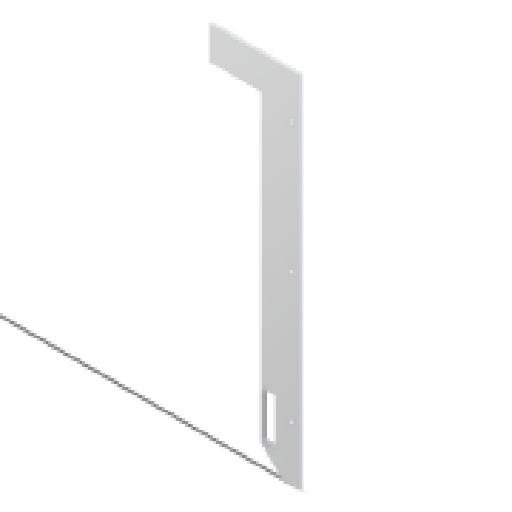
# Autodesk Inventor part: Drag Chain Cover Panel
Saved by Autodesk Inventor 2023.2 (Build 272271000, 271)
## iProperties
Created: 2023-02-24
Part Number: Drag Chain Cover Panel
Material: Aluminum 6061
Document SubType Name: Modeling
Designer: remop
Density: 2.7 g/cm^3
Appearance: Aluminum - Flat
Author: remop
Autodesk Inventor part; units mm, degrees
ref_plane "YZ Plane" through (0, 0, 0) normal (1, 0, 0) x (0, 1, 0)
ref_plane "XZ Plane" through (0, 0, 0) normal (0, 1, 0) x (-1, 0, 0)
ref_plane "XY Plane" through (0, 0, 0) normal (0, 0, 1) x (1, 0, 0)
sketch "Sketch1" plane through (0, 0, 0) normal (0, 0, 1) x (1, 0, 0)
  line L0 (-209.6812, -263.8586) -> (-209.6812, -8.8159) projected
  arc A0 (-209.6812, -8.8159) -> (-193.9694, 2.087) centre (-210.1812, 8.6769) ccw projected
  line L1 (-193.9694, 2.087) -> (-181.7072, 32.2534) projected
  arc A1 (-181.7072, 32.2534) -> (-181.1183, 35.2659) centre (-189.1183, 35.2659) ccw projected
  line L2 (-181.1183, 35.2659) -> (-181.1183, 96.1414) projected
  line L3 (-181.1183, 96.1414) -> (-26.7601, 96.1414) projected
  line L4 (-26.7601, 96.1414) -> (-26.7601, -154.4598) projected
  line L5 (-26.7601, -154.4598) -> (-51.6589, -154.4598) projected
  arc A2 (-51.6589, -154.4598) -> (-66.1514, -181.7688) centre (-51.6589, -171.9598) ccw projected
  line L6 (-66.1514, -181.7688) -> (-37.4983, -224.1032) projected
  line L7 (-37.4983, -224.1032) -> (-37.4983, -263.8586) projected
  line L8 (-37.4983, -263.8586) -> (-209.6812, -263.8586) projected
  circle A3 centre (-14.2602, -188.2205) radius 1.4 projected
  circle A4 centre (7.7398, -188.2205) radius 1.4 projected
  circle A5 centre (-3.2602, -180.2205) radius 1.4 projected
  line L9 (38.5068, -227.443) -> (38.5068, -237.331) projected
  line L10 (38.5068, -237.331) -> (14.3647, -261.4731) projected
  line L11 (14.3647, -261.4731) -> (4.4767, -261.4731) projected
  line L12 (4.4767, -261.4731) -> (-26.5537, -230.4427) projected
  arc A6 (-26.9169, -230.0029) -> (-26.5537, -230.4427) centre (-24.4324, -228.3213) ccw projected
  line L13 (-26.9169, -230.0029) -> (-61.6727, -178.6518) projected
  arc A7 (-44.3145, -161.2936) -> (-61.6727, -178.6518) centre (-51.3209, -171.6454) ccw projected
  line L14 (-44.3145, -161.2936) -> (-22.2602, -176.2205) projected
  line L15 (-22.2602, -176.2205) -> (15.7398, -176.2205) projected
  line L16 (15.7398, -176.2205) -> (15.7398, -204.6759) projected
  line L17 (15.7398, -204.6759) -> (38.5068, -227.443) projected
  circle A8 centre (21.8647, -223.6177) radius 4 projected
  circle A9 centre (0.6515, -202.4045) radius 4 projected
  circle A10 centre (-20.5617, -223.6177) radius 4 projected
  circle A11 centre (0.6515, -244.831) radius 4 projected
  circle A12 centre (0.6515, -223.6177) radius 13 projected
  line L18 (55.2634, 96.1414) -> (55.2634, -263.8586) projected
  line L19 (40.2634, 96.1414) -> (-459.7366, 96.1414) projected
  line L20 (40.2634, 96.1414) -> (55.2634, 96.1414)
  line L21 (20.2634, 66.0678) -> (-26.7366, 66.0678) projected
  line L22 (20.2634, -173.9322) -> (20.2634, 66.0678) projected
  line L23 (20.2634, -173.9322) -> (20.2634, -206.3712)
  line L24 (20.2634, -206.3712) -> (40.2634, -226.3712)
  line L25 (40.2634, -226.3712) -> (55.2634, -226.3712)
  line L26 (-25.7601, 66.0678) -> (-25.7601, 96.1414)
  circle A13 centre (-71.7601, 91.1414) radius 1.45 projected
  circle A14 centre (-41.7601, 91.1414) radius 1.45 projected
  circle A15 centre (-66.4329, -190.3739) radius 1.45 projected
  circle A16 centre (-46.6589, -149.4598) radius 1.45 projected
  circle A17 centre (-195.1812, -258.8586) radius 1.45 projected
  circle A18 centre (-174.1183, 35.2659) radius 1.45 projected
  line L27 (-48.8209, -179.8954) -> (-45.8209, -179.8954) projected
  line L28 (-45.8209, -179.8954) -> (-45.8209, -163.3954) projected
  line L29 (-45.8209, -163.3954) -> (-48.8209, -163.3954) projected
  line L30 (-48.8209, -163.3954) -> (-48.8209, -179.8954) projected
  line L31 (-56.8209, -179.8954) -> (-53.8209, -179.8954) projected
  line L32 (-53.8209, -179.8954) -> (-53.8209, -163.3954) projected
  line L33 (-53.8209, -163.3954) -> (-56.8209, -163.3954) projected
  line L34 (-56.8209, -163.3954) -> (-56.8209, -179.8954) projected
  point P0 (0, 0)
  dimension "d0" = 2
  dimension "d1" = 15
  dimension "d2" = 1
  constraints: 10 end point, 3 point on line, 2 perpendicular, 1 horizontal, 1 parallel, 1 vertical
  measures "d0" distance between parallel lines of L17 L24
  measures "d1" distance of L24.end L25.end
  measures "d2" distance between parallel lines of L4 L26
extrude "Extrusion1" add sketch "Sketch1" along normal blind 3 contours L18 L25 L24 L23 L22 L21 L26 L19 L20
sketch "Sketch2" plane through (0, 0, 0) normal (0, 0, -1) x (-1, 0, 0)
  line L0 (-20.2634, 66.0678) -> (-20.2634, -206.3712) projected
  line L1 (-20.2634, -206.3712) -> (-40.2634, -226.3712) projected
  line L2 (-40.2634, -226.3712) -> (-55.2634, -226.3712) projected
  line L3 (25.7601, 66.0678) -> (-20.2634, 66.0678) projected
  line L4 (25.7601, 96.1414) -> (25.7601, 66.0678) projected
  circle A0 centre (-47.7634, -176.3712) radius 1.75
  circle A1 centre (-47.7634, -60.1149) radius 1.75
  circle A2 centre (-47.7634, 56.1414) radius 1.75
  line L5 (-23.2634, -203.3712) -> (-33.2634, -203.3712)
  line L6 (-33.2634, -203.3712) -> (-33.2634, -163.3712)
  line L7 (-33.2634, -163.3712) -> (-23.2634, -163.3712)
  line L8 (-23.2634, -163.3712) -> (-23.2634, -203.3712)
  point P0 (0, 0)
  dimension "d5" = 7.5
  dimension "d6" = 3.5
  dimension "d7" = 50
  dimension "d8" = 40
  dimension "d9" = 232.5126
  dimension "d10" = 116.2563
  dimension "d11" = 3
  dimension "d12" = 10
  dimension "d13" = 40
  dimension "d14" = 3
  constraints: 8 end point, 3 centre point, 2 equal radius, 2 parallel, 2 vertical alignment, 1 horizontal, 1 perpendicular
  measures "d5" horizontal distance of L2.end A0.centre
  measures "d6" diameter of A0
  measures "d7" distance from line of L2 A0.centre
  measures "d8" vertical distance of L4.start A2.centre
  measures "d9" distance of A0.centre A2.centre
  measures "d10" distance of A2.centre A1.centre
  measures "d11" distance from line of L0 L7.end
  measures "d12" distance of L6.end L7.end
  measures "d13" distance of L7.end L5.start
  measures "d14" distance from line of L0.end L5
extrude "Extrusion2" cut sketch "Sketch2" against normal through all
equation "\"d10\" = 0.5 * d9"
body "Solid1"
